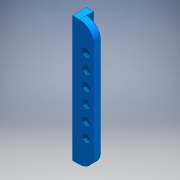
# Autodesk Inventor part: bottomSideFrame
Saved by Autodesk Inventor 2016 (Build 200138000, 138)
## iProperties
Created: 2016-06-05
Part Number: bottomSideFrame
Material: ABS Plastic
Document SubType Name: Modeling
Designer: hesaon
Density: 1.06 g/cm^3
Appearance: Smooth - White
Author: hesaon
Autodesk Inventor part; units mm, degrees
ref_plane "YZ Plane" through (0, 0, 0) normal (1, 0, 0) x (0, 1, 0)
ref_plane "XZ Plane" through (0, 0, 0) normal (0, 1, 0) x (-1, 0, 0)
ref_plane "XY Plane" through (0, 0, 0) normal (0, 0, 1) x (1, 0, 0)
sketch "Sketch1" plane through (0, 0, 0) normal (0, 1, 0) x (-1, 0, 0)
  line L0 (-30, -20) -> (-30, -158)
  line L1 (-10, -178) -> (0, -178)
  line L2 (0, -178) -> (0, 0)
  arc A0 (-10, 0) -> (-30, -20) centre (-10, -20) ccw
  line L3 (-10, -20) -> (-30, -20) construction
  line L4 (-10, -20) -> (-10, 0) construction
  arc A1 (-30, -158) -> (-10, -178) centre (-10, -158) ccw
  line L5 (-10, -158) -> (-10, -178) construction
  line L6 (-10, -158) -> (-30, -158) construction
  line L7 (0, 0) -> (-10, 0)
  dimension "d2" = 90
  dimension "d4" = 10
  dimension "d6" = 90
  dimension "d10" = 20
  dimension "d11" = 20
  dimension "d12" = 178
  dimension "d112" = 20
  dimension "d113" = 10
  constraints: 16 end point, 4 point on circle, 2 centre point, 2 parallel, 1 horizontal, 1 tangent
  measures "d2" angle of L4 L3
  measures "d4" horizontal distance of L3.start L2.end
  measures "d6" angle of L6 L5
  measures "d10" horizontal distance of L4.end L0.start
  measures "d11" horizontal distance of L0.end L1.start
  measures "d12" distance of L1.end L2.end
  measures "d112" distance of L1.start L5.start
  measures "d113" distance of L1.start L1.end
extrude "Extrusion1" add sketch "Sketch1" along normal blind 10
sketch "Sketch3" plane through (0, 10, 0) normal (0, 1, 0) x (1, 0, 0)
  line L0 (0, 0) -> (0, 178) projected
  line L1 (0, 0) -> (10, 0)
  line L2 (10, 0) -> (10, 10)
  line L3 (10, 10) -> (0, 10)
  line L4 (0, 10) -> (0, 0)
  line L5 (0, 178) -> (0, 0) projected
  line L6 (0, 0) -> (10, 0) projected
  line L7 (0, 52) -> (10, 52)
  line L8 (10, 52) -> (10, 62)
  line L9 (10, 62) -> (0, 62)
  line L10 (0, 62) -> (0, 52)
  line L11 (10, 118) -> (0, 118)
  line L12 (0, 118) -> (0, 128)
  line L13 (0, 128) -> (10, 128)
  line L14 (10, 128) -> (10, 118)
  dimension "d39" = 10
  dimension "d40" = 10
  dimension "d41" = 10
  dimension "d42" = 10
  dimension "d43" = 42
  dimension "d44" = 10
  dimension "d45" = 10
  dimension "d46" = 56
  constraints: 24 end point, 6 parallel, 4 collinear, 3 horizontal, 3 perpendicular
  measures "d39" distance of L3.end L2.end
  measures "d40" distance of L2.end L1.end
  measures "d41" distance of L9.end L8.end
  measures "d42" distance of L8.end L7.end
  measures "d43" distance between parallel lines of L7 L3
  measures "d44" distance of L12.end L13.end
  measures "d45" distance of L11.end L12.end
  measures "d46" distance between parallel lines of L9 L11
extrude "Extrusion3" add sketch "Sketch3" along normal blind 10
sketch "Sketch4" plane through (0, 10, 0) normal (0, 1, 0) x (1, 0, 0)
  line L0 (10, 62) -> (0, 62)
  line L1 (0, 62) -> (0, 118)
  line L2 (0, 118) -> (10, 118)
  line L3 (10, 118) -> (10, 62)
  line L4 (10, 62) -> (0, 62) projected
  line L5 (0, 118) -> (10, 118) projected
  line L6 (0, 118) -> (0, 62) projected
  point P0 (0, 0)
  dimension "d49" = 10
  constraints: 8 end point, 3 collinear, 2 parallel, 1 horizontal, 1 perpendicular
  measures "d49" distance of L1.end L2.end
extrude "Extrusion4" add sketch "Sketch4" along normal blind 10
hole "Hole1" at (10, 15, -5) direction (-1, 0, 0) diameter 4.3 end up to surface
hole "Hole2" at (10, 15, -57) direction (-1, 0, 0) diameter 4.3 end up to surface
hole "Hole3" at (10, 15, -123) direction (-1, 0, 0) diameter 4.3 end up to surface
sketch "Sketch6" plane through (0, 10, 0) normal (0, 1, 0) x (1, 0, 0)
  line L0 (0, 168) -> (10, 168)
  line L1 (10, 168) -> (10, 178)
  line L2 (10, 178) -> (0, 178)
  line L3 (0, 178) -> (0, 168)
  line L4 (10, 178) -> (0, 178) projected
  line L5 (0, 178) -> (0, 128) projected
  dimension "d90" = 10
  dimension "d91" = 10
  constraints: 8 end point, 2 collinear, 2 parallel, 1 horizontal, 1 perpendicular
  measures "d90" distance of L2.end L1.end
  measures "d91" distance of L1.end L0.end
extrude "Extrusion6" add sketch "Sketch6" along normal blind 10
hole "Hole4" at (10, 15, -173) direction (-1, 0, 0) diameter 4.3 end up to surface
sketch "Sketch9" plane through (0, 10, 0) normal (0, 1, 0) x (1, 0, 0)
  line L0 (0, 10) -> (10, 10)
  line L1 (10, 10) -> (10, 20)
  line L2 (10, 20) -> (0, 20)
  line L3 (0, 20) -> (0, 10)
  line L4 (0, 52) -> (0, 10) projected
  line L5 (10, 10) -> (0, 10) projected
  line L6 (0, 158) -> (10, 158)
  line L7 (10, 158) -> (10, 168)
  line L8 (10, 168) -> (0, 168)
  line L9 (0, 168) -> (0, 158)
  line L10 (0, 168) -> (0, 128) projected
  line L11 (0, 168) -> (10, 168) projected
  point P0 (0, 0)
  dimension "d115" = 10
  dimension "d116" = 10
  dimension "d117" = 10
  dimension "d118" = 10
  constraints: 16 end point, 4 collinear, 4 parallel, 2 horizontal, 2 perpendicular
  measures "d115" distance of L2.end L1.end
  measures "d116" distance of L1.end L0.end
  measures "d117" distance of L7.end L8.end
  measures "d118" distance of L7.end L6.end
extrude "Extrusion8" add sketch "Sketch9" along normal blind 10
hole "Hole5" at (10, 15, -15) direction (-1, 0, 0) diameter 4.3 end up to surface
hole "Hole6" at (10, 15, -163) direction (-1, 0, 0) diameter 4.3 end up to surface
sketch "Sketch10" plane through (0, 10, 0) normal (0, 1, 0) x (1, 0, 0)
  line L0 (0, 42) -> (10, 42)
  line L1 (10, 42) -> (10, 52)
  line L2 (10, 52) -> (0, 52)
  line L3 (0, 52) -> (0, 42)
  line L4 (0, 52) -> (10, 52) projected
  line L5 (0, 52) -> (0, 20) projected
  line L6 (0, 128) -> (10, 128)
  line L7 (10, 128) -> (10, 138)
  line L8 (10, 138) -> (0, 138)
  line L9 (0, 138) -> (0, 128)
  line L10 (10, 128) -> (0, 128) projected
  line L11 (0, 158) -> (0, 128) projected
  point P0 (0, 0)
  dimension "d139" = 10
  dimension "d140" = 10
  dimension "d141" = 10
  dimension "d142" = 10
  constraints: 16 end point, 4 collinear, 4 parallel, 2 horizontal, 2 perpendicular
  measures "d139" distance of L2.end L1.end
  measures "d140" distance of L1.end L0.end
  measures "d141" distance of L8.end L7.end
  measures "d142" distance of L7.end L6.end
extrude "Extrusion9" add sketch "Sketch10" along normal blind 10
hole "Hole7" at (0, 15, -47) direction (1, 0, 0) diameter 4.3 end up to surface
hole "Hole8" at (0, 15, -133) direction (1, 0, 0) diameter 4.3 end up to surface
sketch "Sketch11" plane through (0, 0, 0) normal (0, -1, 0) x (1, 0, 0)
  circle A0 centre (20, -78.5) radius 3.1
  circle A1 centre (20, -57.5) radius 3.1
  circle A2 centre (20, -36.5) radius 3.1
  circle A3 centre (20, -99.5) radius 3.1
  circle A4 centre (20, -120.5) radius 3.1
  circle A5 centre (20, -141.5) radius 3.1
  line L0 (10, 0) -> (0, 0) projected
  line L1 (30, -158) -> (30, -20) projected
  dimension "d164" = 6.2
  dimension "d165" = 6.2
  dimension "d166" = 6.2
  dimension "d167" = 6.2
  dimension "d168" = 6.2
  dimension "d169" = 21
  dimension "d170" = 6.2
  dimension "d171" = 21
  dimension "d172" = 21
  dimension "d173" = 21
  dimension "d174" = 21
  dimension "d177" = 99.5
  dimension "d178" = 10
  dimension "d180" = 10
  dimension "d181" = 10
  dimension "d182" = 10
  dimension "d183" = 10
  dimension "rh" = 10
  constraints: 6 centre point
  measures "d164" diameter of A0
  measures "d165" diameter of A1
  measures "d166" diameter of A2
  measures "d167" diameter of A3
  measures "d168" diameter of A4
  measures "d169" distance of A0.centre A3.centre
  measures "d170" diameter of A5
  measures "d171" distance of A3.centre A4.centre
  measures "d172" distance of A5.centre A4.centre
  measures "d173" distance of A1.centre A0.centre
  measures "d174" distance of A2.centre A1.centre
  measures "d177" distance from line of L0 A3.centre
  measures "d178" distance from line of L1 A5.centre
  measures "d180" distance from line of L1 A4.centre
  measures "d181" distance from line of L1 A3.centre
  measures "d182" distance from line of L1 A0.centre
  measures "d183" distance from line of L1 A1.centre
  measures "rh" distance from line of L1 A2.centre
extrude "Extrusion10" cut sketch "Sketch11" against normal up to next
sketch "Sketch12" plane through (0, 0, 0) normal (0, -1, 0) x (1, 0, 0)
  circle A0 centre (20, -36.5) radius 3.1 projected
  line L0 (25.2, -39.5022) -> (20, -42.5044)
  line L1 (20, -42.5044) -> (14.8, -39.5022)
  line L2 (14.8, -39.5022) -> (14.8, -33.4978)
  line L3 (14.8, -33.4978) -> (20, -30.4956)
  line L4 (20, -30.4956) -> (25.2, -33.4978)
  line L5 (25.2, -33.4978) -> (25.2, -39.5022)
  circle A1 centre (20, -57.5) radius 3.1 projected
  line L6 (25.2, -60.5022) -> (20, -63.5044)
  line L7 (20, -63.5044) -> (14.8, -60.5022)
  line L8 (14.8, -60.5022) -> (14.8, -54.4978)
  line L9 (14.8, -54.4978) -> (20, -51.4956)
  line L10 (20, -51.4956) -> (25.2, -54.4978)
  line L11 (25.2, -54.4978) -> (25.2, -60.5022)
  circle A2 centre (20, -78.5) radius 3.1 projected
  line L12 (25.2, -81.5022) -> (20, -84.5044)
  line L13 (20, -84.5044) -> (14.8, -81.5022)
  line L14 (14.8, -81.5022) -> (14.8, -75.4978)
  line L15 (14.8, -75.4978) -> (20, -72.4956)
  line L16 (20, -72.4956) -> (25.2, -75.4978)
  line L17 (25.2, -75.4978) -> (25.2, -81.5022)
  circle A3 centre (20, -99.5) radius 3.1 projected
  line L18 (25.2, -102.5022) -> (20, -105.5044)
  line L19 (20, -105.5044) -> (14.8, -102.5022)
  line L20 (14.8, -102.5022) -> (14.8, -96.4978)
  line L21 (14.8, -96.4978) -> (20, -93.4956)
  line L22 (20, -93.4956) -> (25.2, -96.4978)
  line L23 (25.2, -96.4978) -> (25.2, -102.5022)
  circle A4 centre (20, -120.5) radius 3.1 projected
  line L24 (25.2, -123.5022) -> (20, -126.5044)
  line L25 (20, -126.5044) -> (14.8, -123.5022)
  line L26 (14.8, -123.5022) -> (14.8, -117.4978)
  line L27 (14.8, -117.4978) -> (20, -114.4956)
  line L28 (20, -114.4956) -> (25.2, -117.4978)
  line L29 (25.2, -117.4978) -> (25.2, -123.5022)
  circle A5 centre (20, -141.5) radius 3.1 projected
  line L30 (25.2, -144.5022) -> (20, -147.5044)
  line L31 (20, -147.5044) -> (14.8, -144.5022)
  line L32 (14.8, -144.5022) -> (14.8, -138.4978)
  line L33 (14.8, -138.4978) -> (20, -135.4956)
  line L34 (20, -135.4956) -> (25.2, -138.4978)
  line L35 (25.2, -138.4978) -> (25.2, -144.5022)
  point P0 (0, 0)
  point P1 (25.2, -141.5)
  point P2 (25.2, -120.5)
  point P3 (25.2, -99.5)
  point P4 (25.2, -78.5)
  point P5 (25.2, -57.5)
  point P6 (25.2, -36.5)
  dimension "d187" = 10.4
  dimension "d188" = 10.4
  dimension "d189" = 10.4
  dimension "d190" = 10.4
  dimension "d191" = 10.4
  constraints: 72 end point, 6 coincident, 6 midpoint, 6 vertical alignment, 1 point on line, 78 other
  measures "d187" distance between parallel lines of L1 L4
  measures "d188" distance between parallel lines of L7 L10
  measures "d189" distance between parallel lines of L13 L16
  measures "d190" distance between parallel lines of L19 L22
  measures "d191" distance between parallel lines of L31 L34
extrude "Extrusion11" cut sketch "Sketch12" against normal blind 5
sketch "Sketch14" plane through (0, 10, 0) normal (0, 1, 0) x (1, 0, 0)
  line L0 (10, 64.5) -> (15, 64.5)
  line L1 (15, 64.5) -> (15, 71.5)
  line L2 (15, 71.5) -> (10, 71.5)
  line L3 (10, 71.5) -> (10, 64.5)
  line L4 (10, 85.5) -> (15, 85.5)
  line L5 (15, 85.5) -> (15, 92.5)
  line L6 (15, 92.5) -> (10, 92.5)
  line L7 (10, 92.5) -> (10, 85.5)
  line L8 (10, 106.5) -> (15, 106.5)
  line L9 (15, 106.5) -> (15, 113.5)
  line L10 (15, 113.5) -> (10, 113.5)
  line L11 (10, 113.5) -> (10, 106.5)
  line L12 (10, 42) -> (10, 138) projected
  circle A0 centre (20, 120.5) radius 3.1 projected
  circle A1 centre (20, 99.5) radius 3.1 projected
  circle A2 centre (20, 78.5) radius 3.1 projected
  point P0 (0, 0)
  dimension "d200" = 5
  dimension "d201" = 7
  dimension "d202" = 5
  dimension "d203" = 7
  dimension "d204" = 5
  dimension "d205" = 7
  dimension "d206" = 7
  dimension "d207" = 7
  dimension "d208" = 7
  constraints: 24 end point, 6 parallel, 3 collinear, 3 horizontal, 3 perpendicular
  measures "d200" distance of L2.end L1.end
  measures "d201" distance of L1.end L0.end
  measures "d202" distance of L6.end L5.end
  measures "d203" distance of L5.end L4.end
  measures "d204" distance of L10.end L9.end
  measures "d205" distance of L9.end L8.end
  measures "d206" distance from line of A0.centre L10
  measures "d207" distance from line of A1.centre L6
  measures "d208" distance from line of A2.centre L2
extrude "Extrusion12" add sketch "Sketch14" along normal blind 10 contours L3 L2 L1 L0 | L7 L6 L5 L4 | L11 L10 L9 L8
chamfer "Chamfer2" distance 5 distance2 10 1 edges at (15, 20, -68) measured on face at (14.5, 20, -68)
chamfer "Chamfer3" distance 5 distance2 10 1 edges at (15, 20, -110) measured on face at (14.5, 20, -110)
chamfer "Chamfer4" distance 5 distance2 10 1 edges at (15, 20, -89) measured on face at (14.5, 20, -89)
equation "\"d178\" = rh"
equation "\"d180\" = rh"
equation "\"d181\" = rh"
equation "\"d182\" = rh"
equation "\"d183\" = rh"
body "Solid1"
